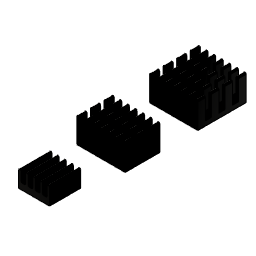
Heat Sinks Pi 4B (Autodesk Fusion 360 design; units mm, degrees)
Autodesk Fusion 360 part; units mm, degrees
note: some values were not read from the file. Set by a fixed rule: which sketch regions a step uses.
sketch "Skizze1" plane through (0, 0, 0) normal (0, 1, 0) x (1, 0, 0)
  line L0 (7, 7) -> (-7, 7)
  line L1 (-7, 7) -> (-7, -7)
  line L2 (-7, -7) -> (7, -7)
  line L3 (7, -7) -> (7, 7)
  line L4 (7, 7) -> (-7, -7) construction
  line L5 (-7, 7) -> (7, -7) construction
  line L6 (-7, 7) -> (-6.25, 7)
  line L7 (-6.25, 7) -> (-6.25, 4.8)
  line L8 (-6.25, 4.8) -> (-7, 4.8)
  line L9 (-7, 4.8) -> (-7, 7)
  line L10 (-4.7917, 7) -> (-4.0417, 7)
  line L11 (-4.0417, 4.8) -> (-4.7917, 4.8)
  line L12 (-4.7917, 4.8) -> (-4.7917, 7)
  line L13 (-4.0417, 7) -> (-4.0417, 4.8)
  line L14 (-2.5833, 7) -> (-1.8333, 7)
  line L15 (-1.8333, 4.8) -> (-2.5833, 4.8)
  line L16 (-2.5833, 4.8) -> (-2.5833, 7)
  line L17 (-1.8333, 7) -> (-1.8333, 4.8)
  line L18 (-0.375, 7) -> (0.375, 7)
  line L19 (0.375, 4.8) -> (-0.375, 4.8)
  line L20 (-0.375, 4.8) -> (-0.375, 7)
  line L21 (0.375, 7) -> (0.375, 4.8)
  line L22 (1.8333, 7) -> (2.5833, 7)
  line L23 (2.5833, 4.8) -> (1.8333, 4.8)
  line L24 (1.8333, 4.8) -> (1.8333, 7)
  line L25 (2.5833, 7) -> (2.5833, 4.8)
  line L26 (4.0417, 7) -> (4.7917, 7)
  line L27 (4.7917, 4.8) -> (4.0417, 4.8)
  line L28 (4.0417, 4.8) -> (4.0417, 7)
  line L29 (4.7917, 7) -> (4.7917, 4.8)
  line L30 (6.25, 7) -> (7, 7)
  line L31 (7, 4.8) -> (6.25, 4.8)
  line L32 (6.25, 4.8) -> (6.25, 7)
  line L33 (7, 7) -> (7, 4.8)
  line L34 (-7, 3.0667) -> (-6.25, 3.0667)
  line L35 (-6.25, 0.8667) -> (-7, 0.8667)
  line L36 (-7, 0.8667) -> (-7, 3.0667)
  line L37 (-6.25, 3.0667) -> (-6.25, 0.8667)
  line L38 (-4.7917, 3.0667) -> (-4.0417, 3.0667)
  line L39 (-4.0417, 0.8667) -> (-4.7917, 0.8667)
  line L40 (-4.7917, 0.8667) -> (-4.7917, 3.0667)
  line L41 (-4.0417, 3.0667) -> (-4.0417, 0.8667)
  line L42 (-2.5833, 3.0667) -> (-1.8333, 3.0667)
  line L43 (-1.8333, 0.8667) -> (-2.5833, 0.8667)
  line L44 (-2.5833, 0.8667) -> (-2.5833, 3.0667)
  line L45 (-1.8333, 3.0667) -> (-1.8333, 0.8667)
  line L46 (-0.375, 3.0667) -> (0.375, 3.0667)
  line L47 (0.375, 0.8667) -> (-0.375, 0.8667)
  line L48 (-0.375, 0.8667) -> (-0.375, 3.0667)
  line L49 (0.375, 3.0667) -> (0.375, 0.8667)
  line L50 (1.8333, 3.0667) -> (2.5833, 3.0667)
  line L51 (2.5833, 0.8667) -> (1.8333, 0.8667)
  line L52 (1.8333, 0.8667) -> (1.8333, 3.0667)
  line L53 (2.5833, 3.0667) -> (2.5833, 0.8667)
  line L54 (4.0417, 3.0667) -> (4.7917, 3.0667)
  line L55 (4.7917, 0.8667) -> (4.0417, 0.8667)
  line L56 (4.0417, 0.8667) -> (4.0417, 3.0667)
  line L57 (4.7917, 3.0667) -> (4.7917, 0.8667)
  line L58 (6.25, 3.0667) -> (7, 3.0667)
  line L59 (7, 0.8667) -> (6.25, 0.8667)
  line L60 (6.25, 0.8667) -> (6.25, 3.0667)
  line L61 (7, 3.0667) -> (7, 0.8667)
  line L62 (-7, -0.8667) -> (-6.25, -0.8667)
  line L63 (-6.25, -3.0667) -> (-7, -3.0667)
  line L64 (-7, -3.0667) -> (-7, -0.8667)
  line L65 (-6.25, -0.8667) -> (-6.25, -3.0667)
  line L66 (-4.7917, -0.8667) -> (-4.0417, -0.8667)
  line L67 (-4.0417, -3.0667) -> (-4.7917, -3.0667)
  line L68 (-4.7917, -3.0667) -> (-4.7917, -0.8667)
  line L69 (-4.0417, -0.8667) -> (-4.0417, -3.0667)
  line L70 (-2.5833, -0.8667) -> (-1.8333, -0.8667)
  line L71 (-1.8333, -3.0667) -> (-2.5833, -3.0667)
  line L72 (-2.5833, -3.0667) -> (-2.5833, -0.8667)
  line L73 (-1.8333, -0.8667) -> (-1.8333, -3.0667)
  line L74 (-0.375, -0.8667) -> (0.375, -0.8667)
  line L75 (0.375, -3.0667) -> (-0.375, -3.0667)
  line L76 (-0.375, -3.0667) -> (-0.375, -0.8667)
  line L77 (0.375, -0.8667) -> (0.375, -3.0667)
  line L78 (1.8333, -0.8667) -> (2.5833, -0.8667)
  line L79 (2.5833, -3.0667) -> (1.8333, -3.0667)
  line L80 (1.8333, -3.0667) -> (1.8333, -0.8667)
  line L81 (2.5833, -0.8667) -> (2.5833, -3.0667)
  line L82 (4.0417, -0.8667) -> (4.7917, -0.8667)
  line L83 (4.7917, -3.0667) -> (4.0417, -3.0667)
  line L84 (4.0417, -3.0667) -> (4.0417, -0.8667)
  line L85 (4.7917, -0.8667) -> (4.7917, -3.0667)
  line L86 (6.25, -0.8667) -> (7, -0.8667)
  line L87 (7, -3.0667) -> (6.25, -3.0667)
  line L88 (6.25, -3.0667) -> (6.25, -0.8667)
  line L89 (7, -0.8667) -> (7, -3.0667)
  line L90 (-7, -4.8) -> (-6.25, -4.8)
  line L91 (-6.25, -7) -> (-7, -7)
  line L92 (-7, -7) -> (-7, -4.8)
  line L93 (-6.25, -4.8) -> (-6.25, -7)
  line L94 (-4.7917, -4.8) -> (-4.0417, -4.8)
  line L95 (-4.0417, -7) -> (-4.7917, -7)
  line L96 (-4.7917, -7) -> (-4.7917, -4.8)
  line L97 (-4.0417, -4.8) -> (-4.0417, -7)
  line L98 (-2.5833, -4.8) -> (-1.8333, -4.8)
  line L99 (-1.8333, -7) -> (-2.5833, -7)
  line L100 (-2.5833, -7) -> (-2.5833, -4.8)
  line L101 (-1.8333, -4.8) -> (-1.8333, -7)
  line L102 (-0.375, -4.8) -> (0.375, -4.8)
  line L103 (0.375, -7) -> (-0.375, -7)
  line L104 (-0.375, -7) -> (-0.375, -4.8)
  line L105 (0.375, -4.8) -> (0.375, -7)
  line L106 (1.8333, -4.8) -> (2.5833, -4.8)
  line L107 (2.5833, -7) -> (1.8333, -7)
  line L108 (1.8333, -7) -> (1.8333, -4.8)
  line L109 (2.5833, -4.8) -> (2.5833, -7)
  line L110 (4.0417, -4.8) -> (4.7917, -4.8)
  line L111 (4.7917, -7) -> (4.0417, -7)
  line L112 (4.0417, -7) -> (4.0417, -4.8)
  line L113 (4.7917, -4.8) -> (4.7917, -7)
  line L114 (6.25, -4.8) -> (7, -4.8)
  line L115 (7, -7) -> (6.25, -7)
  line L116 (6.25, -7) -> (6.25, -4.8)
  line L117 (7, -4.8) -> (7, -7)
  line L118 (-7, -3.0667) -> (7, -3.0667)
  dimension "d1" = 14
  dimension "d2" = 14
  dimension "d3" = 0.75
  dimension "d4" = 2.2
  dimension "d7" = 13.25
  dimension "d8" = -11.8
  constraint horizontal L0
  constraint perpendicular L0 L1
  constraint parallel L0 L2
  constraint parallel L1 L3
  constraint coincident L4 origin
  constraint coincident L5 origin
  constraint horizontal L6
  constraint vertical L7
  constraint horizontal L8
  constraint vertical L9
  measures "d1" distance of L1.end L2.end
  measures "d2" distance of L0.end L1.end
  measures "d3" distance of L0.end L6.end
  measures "d4" distance of L0.end L8.end
extrude "Extrusion1" add sketch "Skizze1" along normal blind 1.3 contours L0 L3 L30 L31 L32 L33 | L0 L1 L3 L7 L8 L11 L12 L13 L15 L16 L17 L19 L20 L21 L23 L24 L25 L27 L28 L29 L31 L32 L34 L35 L37 L58 L59 L60 L62 L65 L66 L68 L69 L70 L72 L73 L74 L76 L77 L78 L80 L81 L82 L84 L85 L86 L88 L118 | L0 L26 L27 L28 L29 | L3 L58 L59 L60 L61 | L0 L22 L23 L24 L25 | L3 L86 L87 L88 L89 L118 | L1 L2 L3 L63 L67 L71 L75 L79 L83 L87 L90 L93 L94 L96 L97 L98 L100 L101 L102 L104 L105 L106 L108 L109 L110 L112 L113 L114 L116 L118 | L0 L18 L19 L20 L21 | L2 L3 L114 L115 L116 L117 | L82 L83 L84 L85 L118 | L0 L14 L15 L16 L17 | L2 L110 L111 L112 L113 | L78 L79 L80 L81 L118 | L0 L10 L11 L12 L13 | L2 L106 L107 L108 L109 | L74 L75 L76 L77 L118 | L0 L1 L6 L7 L8 L9 | L2 L102 L103 L104 L105 | L70 L71 L72 L73 L118 | L1 L34 L35 L36 L37 | L2 L98 L99 L100 L101 | L66 L67 L68 L69 L118 | L1 L62 L63 L64 L65 L118 | L2 L94 L95 L96 L97 | L1 L2 L90 L91 L92 L93 | L38 L39 L40 L41 | L42 L43 L44 L45 | L46 L47 L48 L49 | L50 L51 L52 L53 | L54 L55 L56 L57 makes body 1
extrude "Extrusion2" add sketch "Skizze1" along normal blind 7.5 contours L0 L3 L30 L31 L32 L33 | L0 L26 L27 L28 L29 | L3 L58 L59 L60 L61 | L0 L22 L23 L24 L25 | L3 L86 L87 L88 L89 L118 | L0 L18 L19 L20 L21 | L2 L3 L114 L115 L116 L117 | L82 L83 L84 L85 L118 | L0 L14 L15 L16 L17 | L2 L110 L111 L112 L113 | L78 L79 L80 L81 L118 | L0 L10 L11 L12 L13 | L2 L106 L107 L108 L109 | L74 L75 L76 L77 L118 | L0 L1 L6 L7 L8 L9 | L2 L102 L103 L104 L105 | L70 L71 L72 L73 L118 | L1 L34 L35 L36 L37 | L2 L98 L99 L100 L101 | L66 L67 L68 L69 L118 | L1 L62 L63 L64 L65 L118 | L2 L94 L95 L96 L97 | L1 L2 L90 L91 L92 L93 | L38 L39 L40 L41 | L42 L43 L44 L45 | L46 L47 L48 L49 | L50 L51 L52 L53 | L54 L55 L56 L57 bodies 1
fillet "Abrundung1" radius 0.375 56 edges at (-7, 7.5, -5.9) (-6.25, 7.5, -5.9) (-6.25, 7.5, -1.9667) (-7, 7.5, -1.9667) (-7, 7.5, 1.9667) (-6.25, 7.5, 1.9667) (-6.25, 7.5, 5.9) (-7, 7.5, 5.9) (-4.7917, 7.5, -5.9) (-4.7917, 7.5, -1.9667) (-4.7917, 7.5, 1.9667) (-4.0417, 7.5, -5.9) (-4.0417, 7.5, -1.9667) (-4.0417, 7.5, 1.9667) (-4.0417, 7.5, 5.9) (-4.7917, 7.5, 5.9) (-2.5833, 7.5, 5.9) (-1.8333, 7.5, 5.9) (-1.8333, 7.5, 1.9667) (-2.5833, 7.5, 1.9667) (-2.5833, 7.5, -1.9667) (-1.8333, 7.5, -1.9667) (-2.5833, 7.5, -5.9) (-1.8333, 7.5, -5.9) (-0.375, 7.5, -5.9) (0.375, 7.5, -5.9) (-0.375, 7.5, -1.9667) (0.375, 7.5, -1.9667) (0.375, 7.5, 1.9667) (-0.375, 7.5, 1.9667) (-0.375, 7.5, 5.9) (0.375, 7.5, 5.9) (1.8333, 7.5, 5.9) (1.8333, 7.5, 1.9667) (1.8333, 7.5, -1.9667) (1.8333, 7.5, -5.9) (2.5833, 7.5, -5.9) (2.5833, 7.5, -1.9667) (2.5833, 7.5, 1.9667) (2.5833, 7.5, 5.9) (4.0417, 7.5, 5.9) (4.0417, 7.5, 1.9667) (4.0417, 7.5, -1.9667) (4.0417, 7.5, -5.9) (4.7917, 7.5, -5.9) (4.7917, 7.5, -1.9667) (4.7917, 7.5, 1.9667) (4.7917, 7.5, 5.9) (6.25, 7.5, -5.9) (7, 7.5, -5.9) (6.25, 7.5, -1.9667) (7, 7.5, -1.9667) (6.25, 7.5, 1.9667) (7, 7.5, 1.9667) (7, 7.5, 5.9) (6.25, 7.5, 5.9) on bodies 1
fillet "Abrundung2" radius 0.375 48 edges at (-6.25, 1.3, 5.9) (-6.25, 1.3, 1.9667) (-6.25, 1.3, -1.9667) (-6.25, 1.3, -5.9) (-4.7917, 1.3, 5.9) (-4.7917, 1.3, 1.9667) (-4.7917, 1.3, -5.9) (-4.7917, 1.3, -1.9667) (-2.5833, 1.3, -5.9) (-2.5833, 1.3, -1.9667) (-2.5833, 1.3, 1.9667) (-0.375, 1.3, -5.9) (-0.375, 1.3, -1.9667) (-0.375, 1.3, 1.9667) (1.8333, 1.3, 1.9667) (1.8333, 1.3, -1.9667) (1.8333, 1.3, -5.9) (4.0417, 1.3, -5.9) (4.0417, 1.3, -1.9667) (6.25, 1.3, -5.9) (6.25, 1.3, -1.9667) (6.25, 1.3, 1.9667) (4.0417, 1.3, 1.9667) (-2.5833, 1.3, 5.9) (-0.375, 1.3, 5.9) (1.8333, 1.3, 5.9) (4.0417, 1.3, 5.9) (6.25, 1.3, 5.9) (-4.0417, 1.3, -5.9) (-4.0417, 1.3, -1.9667) (-4.0417, 1.3, 1.9667) (-4.0417, 1.3, 5.9) (-1.8333, 1.3, 5.9) (-1.8333, 1.3, 1.9667) (-1.8333, 1.3, -1.9667) (-1.8333, 1.3, -5.9) (0.375, 1.3, -5.9) (0.375, 1.3, -1.9667) (0.375, 1.3, 1.9667) (0.375, 1.3, 5.9) (2.5833, 1.3, 5.9) (2.5833, 1.3, 1.9667) (2.5833, 1.3, -1.9667) (2.5833, 1.3, -5.9) (4.7917, 1.3, -5.9) (4.7917, 1.3, -1.9667) (4.7917, 1.3, 1.9667) (4.7917, 1.3, 5.9) on bodies 1
extrude "Extrusion3" add sketch "Skizze1" along normal blind 12 separate body contours L1 L2 L3 L63 L67 L71 L75 L79 L83 L87 L90 L93 L94 L96 L97 L98 L100 L101 L102 L104 L105 L106 L108 L109 L110 L112 L113 L114 L116 L118 | L2 L3 L114 L115 L116 L117 | L2 L110 L111 L112 L113 | L2 L106 L107 L108 L109 | L2 L102 L103 L104 L105 | L2 L98 L99 L100 L101 | L2 L94 L95 L96 L97 | L1 L2 L90 L91 L92 L93 makes body 2
copy_body "Körper kopieren/einfügen1" bodies 1 makes body 3
move_body "Heat Sink 14x10" bodies 3 to x (1, 0, 0) y (0, 1, 0) z (0, 0, 1) at (0, 1, 0)
combine "Kombinieren1" operation cut target body 3 tool bodies 2
move_body "Verschieben2" bodies 3 to x (1, 0, 0) y (0, 1, 0) z (0, 0, 1) at (0, -1, 25)
sketch "Skizze2" plane through (0, 0, 0) normal (0, 1, 0) x (1, 0, 0)
  line L0 (4.5, 4.5) -> (-4.5, 4.5)
  line L1 (-4.5, 4.5) -> (-4.5, -4.5)
  line L2 (-4.5, -4.5) -> (4.5, -4.5)
  line L3 (4.5, -4.5) -> (4.5, 4.5)
  line L4 (4.5, 4.5) -> (-4.5, -4.5) construction
  line L5 (-4.5, 4.5) -> (4.5, -4.5) construction
  line L6 (-4.5, 4.5) -> (-3.8, 4.5)
  line L7 (-3.8, 4.5) -> (-3.8, -4.5)
  line L8 (-3.8, -4.5) -> (-4.5, -4.5)
  line L9 (-4.5, -4.5) -> (-4.5, 4.5)
  line L10 (-2.425, 4.5) -> (-1.725, 4.5)
  line L11 (-1.725, -4.5) -> (-2.425, -4.5)
  line L12 (-2.425, -4.5) -> (-2.425, 4.5)
  line L13 (-1.725, 4.5) -> (-1.725, -4.5)
  line L14 (-0.35, 4.5) -> (0.35, 4.5)
  line L15 (0.35, -4.5) -> (-0.35, -4.5)
  line L16 (-0.35, -4.5) -> (-0.35, 4.5)
  line L17 (0.35, 4.5) -> (0.35, -4.5)
  line L18 (1.725, 4.5) -> (2.425, 4.5)
  line L19 (2.425, -4.5) -> (1.725, -4.5)
  line L20 (1.725, -4.5) -> (1.725, 4.5)
  line L21 (2.425, 4.5) -> (2.425, -4.5)
  line L22 (3.8, 4.5) -> (4.5, 4.5)
  line L23 (4.5, -4.5) -> (3.8, -4.5)
  line L24 (3.8, -4.5) -> (3.8, 4.5)
  line L25 (4.5, 4.5) -> (4.5, -4.5)
  dimension "d19" = 9
  dimension "d20" = 9
  dimension "d21" = 0.7
  dimension "d24" = 8.3
  dimension "d25" = 0
  constraint horizontal L0
  constraint perpendicular L0 L1
  constraint parallel L0 L2
  constraint parallel L1 L3
  constraint coincident L4 origin
  constraint coincident L5 origin
  constraint horizontal L6
  constraint vertical L7
  constraint horizontal L8
  constraint vertical L9
  constraint coincident L2 L7.end
  measures "d19" distance of L1.end L2.end
  measures "d20" distance of L0.end L1.end
  measures "d21" distance of L0.end L6.end
extrude "Extrusion4" add sketch "Skizze2" along normal blind 1.8 separate body makes body 4
extrude "Extrusion5" add sketch "Skizze2" along normal blind 5 contours L0 L2 L3 L22 L23 L24 L25 | L0 L2 L18 L19 L20 L21 | L0 L2 L14 L15 L16 L17 | L0 L2 L10 L11 L12 L13 | L0 L1 L2 L6 L7 L8 L9 bodies 4
fillet "Abrundung3" radius 0.35 10 edges at (-4.5, 5, 0) (-3.8, 5, 0) (-2.425, 5, 0) (-1.725, 5, 0) (-0.35, 5, 0) (0.35, 5, 0) (1.725, 5, 0) (2.425, 5, 0) (3.8, 5, 0) (4.5, 5, 0) on bodies 4
fillet "Abrundung4" radius 0.35 8 edges at (-3.8, 1.8, 0) (-1.725, 1.8, 0) (0.35, 1.8, 0) (2.425, 1.8, 0) (3.8, 1.8, 0) (1.725, 1.8, 0) (-0.35, 1.8, 0) (-2.425, 1.8, 0) on bodies 4
move_body "Verschieben3" bodies 4 to x (1, 0, 0) y (0, 1, 0) z (0, 0, 1) at (0, 0, 43)
copy_body "Körper->Berechn1" bodies 1 removing the originals makes body 5 in component "Heat Sink 14x14"
copy_body "Körper->Berechn2" bodies 3 removing the originals makes body 6 in component "Heat Sink 14x10"
copy_body "Körper->Berechn3" bodies 4 removing the originals makes body 7 in component "Heat Sink 9x9"
component "Heat Sink 14x14" placed x (1, 0, 0) y (0, 1, 0) z (0, 0, 1) at (0, 0, 0)
component "Heat Sink 14x10" placed x (1, 0, 0) y (0, 1, 0) z (0, 0, 1) at (0, 0, 0)
component "Heat Sink 9x9" placed x (1, 0, 0) y (0, 1, 0) z (0, 0, 1) at (0, 0, 0)
named bodies: "Heat Sink 14x14", "Heat Sink 14x10", "Heat Sink 9x9"
